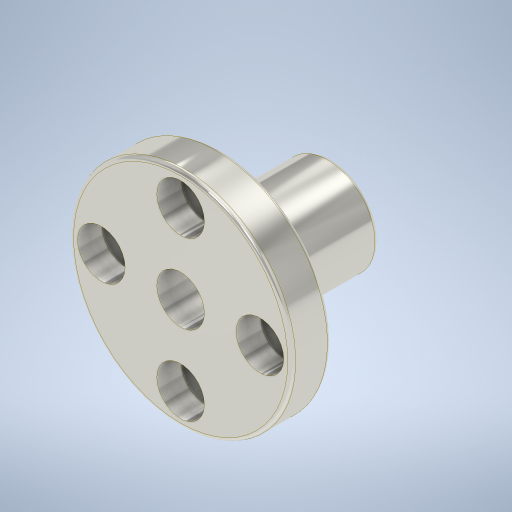
# Autodesk Inventor part: 2309HCMUTE-CDT23-BAC_TRUOT
Saved by Autodesk Inventor 2023 (Build 270158000, 158)
## iProperties
Created: 2023-10-21
Part Number: 2309HCMUTE-CDT23-BAC_TRUOT
Material: Stainless Steel
Document SubType Name: Modeling
Designer: havie
Density: 8 g/cm^3
Appearance: Silver
Author: havie
Autodesk Inventor part; units mm, degrees
ref_plane "YZ Plane" through (0, 0, 0) normal (1, 0, 0) x (0, 1, 0)
ref_plane "XZ Plane" through (0, 0, 0) normal (0, 1, 0) x (-1, 0, 0)
ref_plane "XY Plane" through (0, 0, 0) normal (0, 0, 1) x (1, 0, 0)
sketch "Sketch1" plane through (0, 0, 0) normal (0, 1, 0) x (-1, 0, 0)
  circle A0 centre (0, 0) radius 14
  dimension "d0" = 28
  constraints: 1 centre point, 1 coincident
  measures "d0" diameter of A0
extrude "Extrusion1" add sketch "Sketch1" along normal blind 5
sketch "Sketch2" plane through (0, 5, 0) normal (0, 1, 0) x (1, 0, 0)
  circle A0 centre (0, 0) radius 6
  dimension "d3" = 12
  constraints: 1 centre point, 1 coincident
  measures "d3" diameter of A0
extrude "Extrusion2" add sketch "Sketch2" along normal blind 14
sketch "Sketch4" plane through (0, 0, 0) normal (0, -1, 0) x (1, 0, 0)
  circle A0 centre (0, 0) radius 10 construction
  point P0 (0, -10)
  point P1 (0, 10)
  point P2 (-10, 0)
  point P3 (10, 0)
  dimension "d7" = 20
  constraints: 4 point on circle, 2 horizontal alignment, 2 vertical alignment, 1 centre point, 1 coincident
  measures "d7" diameter of A0
hole "Hole1" at (0, 0, -10) at (0, 0, 10) at (-10, 0, 0) at (10, 0, 0) direction (0, 1, 0) diameter 2.85 end through all counterbore diameter 6 counterbore depth 3.1 thread size "M3.5x0.6" class "6H" standard "ISO Metric profile"
sketch "Sketch5" plane through (0, 19, 0) normal (0, 1, 0) x (1, 0, 0)
  point P0 (0, 0)
  point P1 (0, 0)
  dimension "d6" = 20
  constraints: 1 coincident
hole "Hole2" at (0, 19, 0) direction (0, -1, 0) diameter 6 end through all
fillet "Fillet1" radius 0.5 3 edges at (-6, 19, 0) (14, 5, 0) (14, 0, 0)
body "Solid1"
